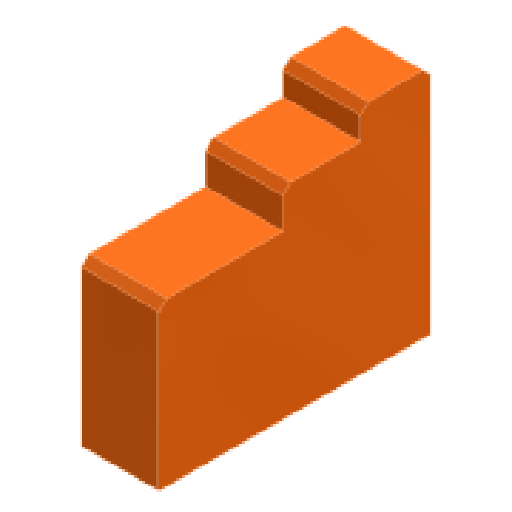
# Autodesk Inventor part: GRJ-05-102
Saved by Autodesk Inventor 2026.1 (Build 301233000, 233)
## iProperties
Created: 2025-08-13
Part Number: GRJ-05-102
Material: Fenolite OR
Document SubType Name: Modeling
Designer: Willian Pinheiro
Density: 1.38 g/cm^3
Appearance: Suave - Laranja claro
Description: Suporte Dissipador
Mass: 9.36398 g
Surface Area: 29.0341 cm^2
Volume: 6.7855 cm^3
Total: 2
Dimensões: 10 x 30 x 35 mm
Author: Willian Pinheiro
Revision Number: 00
Autodesk Inventor part; units mm, degrees
ref_plane "YZ Plane" through (0, 0, 0) normal (1, 0, 0) x (0, 1, 0)
ref_plane "XZ Plane" through (0, 0, 0) normal (0, 1, 0) x (-1, 0, 0)
ref_plane "XY Plane" through (0, 0, 0) normal (0, 0, 1) x (1, 0, 0)
sketch "Esboço1" plane through (0, 0, 0) normal (1, 0, 0) x (0, 1, 0)
  line L0 (-24.5, 0) -> (24.5, 0) construction
  line L1 (0, -21) -> (0, 21) construction
  line L2 (-17.5, 15) -> (17.5, 15)
  line L3 (17.5, 15) -> (17.5, -15)
  line L4 (17.5, -15) -> (-17.5, -15)
  line L5 (-17.5, -15) -> (-17.5, 15)
  line L6 (-17.5, 15) -> (-1.5, 15)
  line L7 (-1.5, 15) -> (-1.5, 6)
  line L8 (-1.5, 6) -> (-17.5, 6)
  line L9 (-17.5, 6) -> (-17.5, 15)
  line L10 (-1.5, 15) -> (8.5, 15)
  line L11 (8.5, 15) -> (8.5, 11)
  line L12 (8.5, 11) -> (-1.5, 11)
  line L13 (-1.5, 11) -> (-1.5, 15)
  point P0 (0, 0)
  point P1 (8.5, 15)
  point P2 (-1.5, 11)
  point P3 (-17.5, 6)
  dimension "d0" = 35
  dimension "d1" = 30
  dimension "d3" = 16
  dimension "d5" = 10
  dimension "d16" = 4
  dimension "d17" = 9
  constraints: 24 end point, 6 parallel, 3 horizontal, 3 perpendicular, 2 other
  measures "d0" distance between parallel lines of L3 L5
  measures "d1" distance between parallel lines of L2 L4
  measures "d3" distance between parallel lines of L5 L7
  measures "d5" distance between parallel lines of L7 L11
  measures "d16" distance between parallel lines of L12 L2
  measures "d17" distance between parallel lines of L8 L2
extrude "Extrusão1" add sketch "Esboço1" along normal mid plane 10 contours L8 L7 L12 L11 L2 L3 L4 L5
sketch "Esboço2" plane through (5, 17.5, -15) normal (0, 0, -1) x (-1, 0, 0)
  point P0 (5, -17.5)
hole "Furo1" at (0, 0, -15) direction (0, 0, 1) diameter 3.242 depth 15 tip angle 118 thread size "M4x0.7" class "6H" standard "ISO Metric profile"
chamfer "Chanfro1" distance 1 angle 45 4 edges at (0, -1.5, 11) (0, 8.5, 15) (0, 17.5, 15) (0, -17.5, 6)
